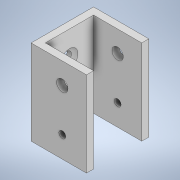
# Autodesk Inventor part: Silder Mount V1
Saved by Autodesk Inventor 2020 (Build 240168000, 168)
## iProperties
Created: 2020-01-20
Part Number: Silder Mount V1
Material: Generic
Document SubType Name: Modeling
Designer: maple
Density: 1 g/cm^3
Appearance: Default
Author: maple
Autodesk Inventor part; units mm, degrees
ref_plane "YZ Plane" through (0, 0, 0) normal (1, 0, 0) x (0, 1, 0)
ref_plane "XZ Plane" through (0, 0, 0) normal (0, 1, 0) x (-1, 0, 0)
ref_plane "XY Plane" through (0, 0, 0) normal (0, 0, 1) x (1, 0, 0)
sketch "Sketch1" plane through (0, 0, 0) normal (0, 1, 0) x (-1, 0, 0)
  line L0 (0, 0) -> (-21.59, 0)
  line L1 (-21.59, 0) -> (-21.59, -21.59)
  line L2 (-21.59, -21.59) -> (0, -21.59)
  line L3 (0, -21.59) -> (0, 0)
  line L4 (-21.59, 0) -> (0, 0)
  line L5 (0, 0) -> (0, 3.175)
  line L6 (0, 3.175) -> (-21.59, 3.175)
  line L7 (-21.59, 3.175) -> (-21.59, 0)
  line L8 (0, 3.175) -> (3.175, 3.175)
  line L9 (3.175, 3.175) -> (3.175, -21.59)
  line L10 (3.175, -21.59) -> (0, -21.59)
  line L11 (0, -21.59) -> (0, 3.175)
  line L12 (3.175, -21.59) -> (-21.59, -21.59)
  line L13 (-21.59, -21.59) -> (-21.59, -24.765)
  line L14 (-21.59, -24.765) -> (3.175, -24.765)
  line L15 (3.175, -24.765) -> (3.175, -21.59)
  dimension "d0" = 21.59
  dimension "d1" = 21.59
  dimension "d2" = 3.175
  dimension "d3" = 3.175
  constraints: 32 end point, 8 parallel, 4 horizontal, 4 perpendicular, 1 point on line
  measures "d0" distance of L2.end L1.end
  measures "d1" distance of L1.end L0.end
  measures "d2" distance of L13.end L12.end
  measures "d3" distance between parallel lines of L3 L9
extrude "Extrusion1" add sketch "Sketch1" along normal blind 38.1 contours L5 L8 L9 L10 L3 | L0 L7 L6 L5 | L10 L15 L14 L13 L2
sketch "Sketch2" plane through (0, 0, 0) normal (1, 0, 0) x (0, 0, -1)
  line L0 (0, 0) -> (21.59, 0) projected
  line L1 (10.795, 0) -> (10.795, 11.43)
  line L2 (10.795, 0) -> (22.225, 0) construction
  line L3 (0, 38.1) -> (21.59, 38.1) projected
  line L4 (10.795, 38.1) -> (10.795, 26.67)
  line L5 (10.795, 38.1) -> (22.225, 38.1) construction
  circle A0 centre (10.795, 26.67) radius 2.159
  circle A1 centre (10.795, 11.43) radius 2.159
  dimension "d6" = 11.43
  dimension "d7" = 90
  dimension "d8" = 11.43
  dimension "d9" = 90
  dimension "d10" = 15.24
  dimension "d11" = 4.318
  dimension "d12" = 4.318
  constraints: 8 end point, 2 centre point, 2 coincident, 2 horizontal, 2 midpoint, 2 perpendicular, 2 vertical
  measures "d6" distance of L1.start L1.end
  measures "d7" angle of L2 L1
  measures "d8" distance of L4.start L4.end
  measures "d9" angle of L4 L5
  measures "d10" distance of L4.end L1.end
  measures "d11" diameter of A0
  measures "d12" diameter of A1
hole "Hole1" at (0, 26.67, -10.795) at (0, 11.43, -10.795) direction (-1, 0, 0) diameter 4.318 depth 26.67 counterbore diameter 7.62 counterbore depth 1.27
sketch "Sketch3" plane through (-3.175, 0, 3.175) normal (0, 0, 1) x (1, 0, 0)
  line L0 (3.175, 38.1) -> (24.765, 38.1) projected
  line L1 (13.97, 38.1) -> (13.97, 28.575)
  circle A0 centre (13.97, 28.575) radius 2.54
  point P0 (3.175, 0)
  dimension "d20" = 9.525
  dimension "d21" = 5.08
  constraints: 2 end point, 1 centre point, 1 coincident, 1 midpoint, 1 vertical
  measures "d20" distance of L1.start L1.end
  measures "d21" diameter of A0
extrude "Extrusion2" cut sketch "Sketch3" against normal blind 38.1
fillet "Fillet1" radius 3.175 2 edges at (-1.27, 11.43, -6.985) (-1.27, 26.67, -6.985)
sketch "Sketch4" plane through (-3.175, 0, 3.175) normal (0, 0, 1) x (1, 0, 0)
  line L0 (24.765, 0) -> (3.175, 0) projected
  line L1 (13.97, 0) -> (13.97, 9.525)
  circle A0 centre (13.97, 9.525) radius 1.524
  dimension "d25" = 9.525
  dimension "d26" = 3.048
  constraints: 2 end point, 1 centre point, 1 coincident, 1 midpoint, 1 vertical
  measures "d25" distance of L1.start L1.end
  measures "d26" diameter of A0
extrude "Extrusion3" cut sketch "Sketch4" against normal blind 38.1
body "Solid1"
